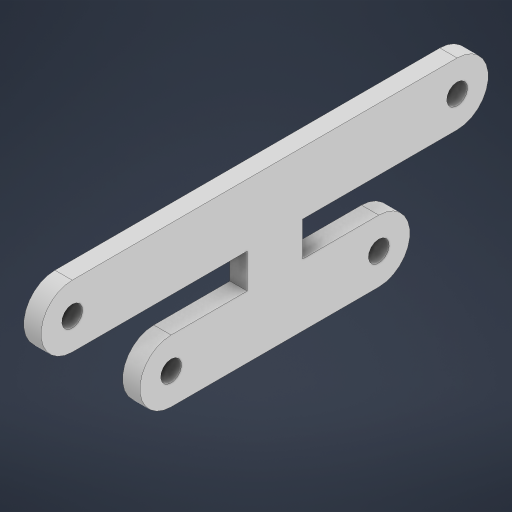
# Autodesk Inventor part: acople_acr
Saved by Autodesk Inventor 2023.1 (Build 271208000, 208)
## iProperties
Created: 2022-10-23
Part Number: acople_acr
Material: Generic
Document SubType Name: Modeling
Designer: amtat
Density: 1 g/cm^3
Appearance: Default
Author: amtat
Autodesk Inventor part; units mm, degrees
ref_plane "YZ Plane" through (0, 0, 0) normal (1, 0, 0) x (0, 1, 0)
ref_plane "XZ Plane" through (0, 0, 0) normal (0, 1, 0) x (-1, 0, 0)
ref_plane "XY Plane" through (0, 0, 0) normal (0, 0, 1) x (1, 0, 0)
sketch "Sketch1" plane through (0, 0, 0) normal (1, 0, 0) x (0, 1, 0)
  circle A0 centre (0, 0) radius 1.5
  line L0 (0, 0) -> (0, -30)
  circle A1 centre (0, -30) radius 1.5
  arc A2 (-4.5, -30) -> (0, -25.5) centre (0, -30) ccw
  arc A3 (4.5, 0) -> (0, -4.5) centre (0, 0) ccw
  line L1 (4.5, 0) -> (4.5, -30)
  line L2 (-4.5, 0) -> (-4.5, -30)
  line L3 (4.5, 0) -> (4.5, -15)
  line L4 (4.5, -15) -> (4.5, -19)
  line L5 (4.5, -15) -> (4.5, -11)
  line L6 (4.5, -11) -> (9.5, -11)
  line L7 (4.5, -19) -> (9.5, -19)
  line L8 (9.5, -11) -> (9.5, -19)
  line L9 (9.5, -19) -> (9.5, -15)
  line L10 (9.5, -15) -> (14, -15)
  line L11 (14, -15) -> (14, -65)
  line L12 (0, 0) -> (14, 14.2829)
  circle A4 centre (14, 14.2829) radius 1.5
  circle A5 centre (14, 14.2829) radius 4.5
  line L13 (14, -15) -> (14, 15.7829)
  line L14 (14, 18.7829) -> (14, 35)
  line L15 (9.5, 14.2829) -> (9.5, -11)
  line L16 (0, -30) -> (14, -41.3137)
  circle A6 centre (14, -41.3137) radius 1.5
  circle A7 centre (14, -41.3137) radius 4.5
  line L17 (9.5, -19) -> (9.5, -41.3137)
  line L18 (18.5, -41.3137) -> (18.5, 14.2829)
  dimension "d15" = 3
  dimension "d0" = 3
  dimension "d1" = 30
  dimension "d2" = 3
  dimension "d3" = 9
  dimension "d4" = 9
  dimension "d5" = 15
  dimension "d6" = 4
  dimension "d7" = 4
  dimension "d8" = 5
  dimension "d9" = 5
  dimension "d10" = 4
  dimension "d11" = 4.5
  dimension "d12" = 50
  dimension "d13" = 50
  dimension "d14" = 20
  dimension "d16" = 9
  dimension "d17" = 18
  dimension "d18" = 3
  dimension "d19" = 9
  constraints: 38 end point, 11 point on circle, 8 coincident, 7 centre point, 6 perpendicular, 6 point on line, 5 tangent, 3 vertical, 2 midpoint, 1 vertical alignment, 2 other
  measures "d0" diameter of A0
  measures "d1" distance of L0.start L0.end
  measures "d2" diameter of A1
  measures "d3" diameter of A2
  measures "d4" diameter of A3
  measures "d5" distance of L1.start L3.end
  measures "d6" distance of L3.end L4.end
  measures "d7" distance of L3.end L5.end
  measures "d8" distance of L5.end L6.end
  measures "d9" distance of L4.end L7.end
  measures "d10" distance of L7.end L9.end
  measures "d11" distance of L9.end L10.end
  measures "d12" distance of L10.end L11.end
  measures "d13" distance of L10.end L14.end
  measures "d14" distance of L12.start L12.end
  measures "d16" diameter of A5
  measures "d17" distance of L16.start L16.end
  measures "d18" diameter of A6
  measures "d19" diameter of A7
extrude "Extrusion1" add sketch "Sketch1" along normal blind 2.5 contours A0 L12 A3 L1 A2 L0 | A0 L0 A3 L12 | L0 A1 L16 A2 L2 A3 | L15 A5 L12 | L12 A5 L13 L10 L8 L15 | A2 L16 A1 L0 | L6 L8 L7 L1 | A5 L13 A4 L12 | L12 A4 L13 A5 | A5 L18 A7 L11 L13 | L10 L11 A7 L16 L17 L8 | L16 A7 L17 | A7 L11 A6 L16 | L16 A6 L11 A7 | A7 L11 A6
body "Solid1"
